Autodesk Inventor part; units mm, degrees
(part 2 of 5)
  arc A499 (38.985, 21.0742) -> (38.8363, 21.0784) centre (38.8363, 18.4135) ccw
  arc A500 (38.8363, 21.0784) -> (38.6875, 21.0742) centre (38.8363, 18.4135) ccw
  arc A501 (38.6875, 21.0742) -> (38.615, 21.0567) centre (38.6991, 20.8676) ccw
  arc A502 (38.615, 21.0567) -> (38.5792, 21.0205) centre (38.6435, 20.9926) ccw
  arc A503 (38.5792, 21.0205) -> (38.5663, 20.9584) centre (38.7225, 20.9584) ccw
  arc A504 (39.9268, 20.274) -> (39.9463, 20.2984) centre (39.9213, 20.2984) ccw
  arc A505 (39.8254, 20.2555) -> (39.9268, 20.274) centre (39.6443, 21.5339) ccw
  arc A506 (39.6897, 20.2426) -> (39.8254, 20.2555) centre (39.615, 21.7404) ccw
  arc A507 (39.5227, 20.2384) -> (39.6897, 20.2426) centre (39.5227, 23.5919) ccw
  arc A508 (39.3451, 20.242) -> (39.5227, 20.2384) centre (39.5227, 24.5793) ccw
  arc A509 (39.2206, 20.2542) -> (39.3451, 20.242) centre (39.3904, 21.3478) ccw
  arc A510 (39.1454, 20.2728) -> (39.2206, 20.2542) centre (39.2876, 20.686) ccw
  arc A511 (39.1363, 20.2984) -> (39.1454, 20.2728) centre (39.1511, 20.2893) ccw
  arc A512 (39.1697, 20.322) -> (39.1363, 20.2984) centre (39.1806, 20.271) ccw
  arc A513 (39.276, 20.3408) -> (39.1697, 20.322) centre (39.4953, 18.7927) ccw
  arc A514 (39.4091, 20.354) -> (39.276, 20.3408) centre (39.5025, 18.7417) ccw
  arc A515 (39.5598, 20.3584) -> (39.4091, 20.354) centre (39.5598, 17.7532) ccw
  arc A516 (39.7105, 20.3542) -> (39.5598, 20.3584) centre (39.5598, 17.6734) ccw
  arc A517 (39.8347, 20.3411) -> (39.7105, 20.3542) centre (39.6388, 19.0798) ccw
  arc A518 (39.9275, 20.3224) -> (39.8347, 20.3411) centre (39.6713, 19.289) ccw
  arc A519 (39.9463, 20.2984) -> (39.9275, 20.3224) centre (39.9216, 20.2984) ccw
  arc A520 (40.3232, 19.7911) -> (40.3363, 19.8184) centre (40.321, 19.8089) ccw
  arc A521 (40.1463, 19.7738) -> (40.3232, 19.7911) centre (39.8685, 23.525) ccw
  arc A522 (39.8917, 19.7619) -> (40.1463, 19.7738) centre (39.8016, 24.4273) ccw
  arc A523 (39.5263, 19.7584) -> (39.8917, 19.7619) centre (39.5263, 38.6953) ccw
  arc A524 (39.1609, 19.7619) -> (39.5263, 19.7584) centre (39.5263, 38.6953) ccw
  arc A525 (38.9062, 19.7738) -> (39.1609, 19.7619) centre (39.2509, 24.4273) ccw
  arc A526 (38.7294, 19.7911) -> (38.9062, 19.7738) centre (39.1841, 23.525) ccw
  arc A527 (38.7163, 19.8184) -> (38.7294, 19.7911) centre (38.7316, 19.8089) ccw
  arc A528 (38.7565, 19.8436) -> (38.7163, 19.8184) centre (38.7619, 19.7902) ccw
  arc A529 (38.9604, 19.8615) -> (38.7565, 19.8436) centre (39.5077, 12.4733) ccw
  arc A530 (39.2151, 19.8743) -> (38.9604, 19.8615) centre (39.3564, 14.5165) ccw
  arc A531 (39.5263, 19.8784) -> (39.2151, 19.8743) centre (39.5263, 8.073) ccw
  arc A532 (39.8375, 19.8743) -> (39.5263, 19.8784) centre (39.5263, 8.073) ccw
  arc A533 (40.0921, 19.8615) -> (39.8375, 19.8743) centre (39.6962, 14.5165) ccw
  arc A534 (40.2961, 19.8436) -> (40.0921, 19.8615) centre (39.5449, 12.4733) ccw
  arc A535 (40.3363, 19.8184) -> (40.2961, 19.8436) centre (40.2906, 19.7902) ccw
  arc A536 (40.3422, 19.3718) -> (40.3663, 19.3984) centre (40.3395, 19.3984) ccw
  arc A537 (40.1413, 19.3545) -> (40.3422, 19.3718) centre (39.6532, 26.1878) ccw
  arc A538 (39.8773, 19.3422) -> (40.1413, 19.3545) centre (39.7622, 24.661) ccw
  arc A539 (39.5263, 19.3384) -> (39.8773, 19.3422) centre (39.5263, 35.57) ccw
  arc A540 (39.1753, 19.3422) -> (39.5263, 19.3384) centre (39.5263, 35.57) ccw
  arc A541 (38.9113, 19.3545) -> (39.1753, 19.3422) centre (39.2903, 24.661) ccw
  arc A542 (38.7103, 19.3718) -> (38.9113, 19.3545) centre (39.3994, 26.1878) ccw
  arc A543 (38.6863, 19.3984) -> (38.7103, 19.3718) centre (38.713, 19.3984) ccw
  arc A544 (38.7103, 19.425) -> (38.6863, 19.3984) centre (38.713, 19.3984) ccw
  arc A545 (38.9113, 19.4423) -> (38.7103, 19.425) centre (39.3994, 12.609) ccw
  arc A546 (39.1753, 19.4546) -> (38.9113, 19.4423) centre (39.2903, 14.1358) ccw
  arc A547 (39.5263, 19.4584) -> (39.1753, 19.4546) centre (39.5263, 3.2268) ccw
  arc A548 (39.8773, 19.4546) -> (39.5263, 19.4584) centre (39.5263, 3.2268) ccw
  arc A549 (40.1413, 19.4423) -> (39.8773, 19.4546) centre (39.7622, 14.1358) ccw
  arc A550 (40.3422, 19.425) -> (40.1413, 19.4423) centre (39.6532, 12.609) ccw
  arc A551 (40.3663, 19.3984) -> (40.3422, 19.425) centre (40.3395, 19.3984) ccw
  arc A552 (39.1063, 18.1289) -> (39.0042, 18.0292) centre (40.3844, 16.7178) ccw
  arc A553 (39.0042, 18.0292) -> (38.9208, 17.9318) centre (39.9041, 17.1742) ccw
  arc A554 (38.9208, 17.9318) -> (38.862, 17.8473) centre (39.7541, 17.2897) ccw
  arc A555 (38.862, 17.8473) -> (38.8539, 17.8014) centre (38.9148, 17.8143) ccw
  arc A556 (38.8534, 17.7698) -> (38.8539, 17.8014) centre (38.7843, 17.7866) ccw
  arc A557 (38.8391, 17.7428) -> (38.8534, 17.7698) centre (38.793, 17.7845) ccw
  arc A558 (38.8129, 17.7247) -> (38.8391, 17.7428) centre (38.7881, 17.7889) ccw
  arc A559 (38.7789, 17.7184) -> (38.8129, 17.7247) centre (38.7789, 17.8128) ccw
  arc A560 (38.7349, 17.7356) -> (38.7789, 17.7184) centre (38.7789, 17.7833) ccw
  arc A561 (38.706, 17.7813) -> (38.7349, 17.7356) centre (38.806, 17.8126) ccw
  arc A562 (38.6904, 17.8667) -> (38.706, 17.7813) centre (39.0419, 17.8865) ccw
  arc A563 (38.6863, 18.014) -> (38.6904, 17.8667) centre (41.3006, 18.014) ccw
  arc A564 (38.6863, 18.014) -> (38.6816, 18.1645) centre (36.253, 18.014) ccw
  arc A565 (38.6816, 18.1645) -> (38.6646, 18.2541) centre (38.3197, 18.142) ccw
  arc A566 (38.6646, 18.2541) -> (38.6322, 18.3075) centre (38.5347, 18.2119) ccw
  arc A567 (38.6322, 18.3075) -> (38.5813, 18.337) centre (38.5534, 18.2302) ccw
  arc A568 (38.5813, 18.3478) -> (38.5813, 18.337) centre (38.5827, 18.3424) ccw
  arc A569 (38.6393, 18.3577) -> (38.5813, 18.3478) centre (38.6742, 17.9809) ccw
  arc A570 (38.7603, 18.3654) -> (38.6393, 18.3577) centre (38.8295, 16.3032) ccw
  arc A571 (38.9263, 18.369) -> (38.7603, 18.3654) centre (38.9968, 11.3177) ccw
  line L156 (38.9263, 18.369) -> (39.3763, 18.3735)
  line L157 (39.3763, 18.3735) -> (39.1063, 18.1289)
  arc A572 (40.71, 17.8434) -> (40.7396, 18.1384) centre (33.6679, 18.699) ccw
  arc A573 (40.6701, 17.7276) -> (40.71, 17.8434) centre (40.4206, 17.8785) ccw
  arc A574 (40.5987, 17.6831) -> (40.6701, 17.7276) centre (40.5905, 17.7757) ccw
  arc A575 (40.4691, 17.6911) -> (40.5987, 17.6831) centre (40.5604, 18.1178) ccw
  arc A576 (40.3093, 17.7285) -> (40.4691, 17.6911) centre (41.3948, 22.0136) ccw
  arc A577 (40.2608, 17.7568) -> (40.3093, 17.7285) centre (40.3342, 17.8266) ccw
  arc A578 (40.2559, 17.7953) -> (40.2608, 17.7568) centre (40.2846, 17.7794) ccw
  arc A579 (40.3036, 17.8651) -> (40.2559, 17.7953) centre (40.6516, 17.5763) ccw
  arc A580 (40.3036, 17.8651) -> (40.3314, 17.916) centre (40.1868, 17.962) ccw
  arc A581 (40.3314, 17.916) -> (40.3249, 17.9568) centre (40.2875, 17.9299) ccw
  arc A582 (40.3249, 17.9568) -> (40.2792, 17.9975) centre (40.2111, 17.875) ccw
  arc A583 (40.2792, 17.9975) -> (40.1665, 18.0556) centre (39.2902, 16.2179) ccw
  arc A584 (40.0747, 18.1066) -> (40.1665, 18.0556) centre (40.5332, 18.8245) ccw
  arc A585 (40.0105, 18.1596) -> (40.0747, 18.1066) centre (40.2585, 18.3945) ccw
  arc A586 (39.9736, 18.2142) -> (40.0105, 18.1596) centre (40.157, 18.2983) ccw
  arc A587 (39.9636, 18.2699) -> (39.9736, 18.2142) centre (40.0765, 18.2614) ccw
  arc A588 (39.9862, 18.329) -> (39.9636, 18.2699) centre (40.0742, 18.2615) ccw
  arc A589 (40.0362, 18.3614) -> (39.9862, 18.329) centre (40.057, 18.2747) ccw
  arc A590 (40.1372, 18.3726) -> (40.0362, 18.3614) centre (40.1311, 17.9654) ccw
  arc A591 (40.3642, 18.3658) -> (40.1372, 18.3726) centre (40.0207, 10.6454) ccw
  line L158 (40.3642, 18.3658) -> (40.7563, 18.3484)
  line L159 (40.7563, 18.3484) -> (40.7396, 18.1384)
  arc A592 (39.7374, 17.7553) -> (39.7363, 17.7784) centre (39.716, 17.7659) ccw
  arc A593 (39.7177, 17.7356) -> (39.7374, 17.7553) centre (39.6982, 17.7747) ccw
  arc A594 (39.6756, 17.7225) -> (39.7177, 17.7356) centre (39.6568, 17.8575) ccw
  arc A595 (39.6163, 17.7184) -> (39.6756, 17.7225) centre (39.6163, 18.149) ccw
  arc A596 (39.557, 17.7225) -> (39.6163, 17.7184) centre (39.6163, 18.149) ccw
  arc A597 (39.5148, 17.7356) -> (39.557, 17.7225) centre (39.5758, 17.8575) ccw
  arc A598 (39.4952, 17.7553) -> (39.5148, 17.7356) centre (39.5344, 17.7747) ccw
  arc A599 (39.4963, 17.7784) -> (39.4952, 17.7553) centre (39.5166, 17.7659) ccw
  arc A600 (39.5166, 17.8014) -> (39.4963, 17.7784) centre (39.5733, 17.7308) ccw
  arc A601 (39.5468, 17.8208) -> (39.5166, 17.8014) centre (39.6223, 17.6699) ccw
  arc A602 (39.5818, 17.8339) -> (39.5468, 17.8208) centre (39.6278, 17.6589) ccw
  arc A603 (39.6163, 17.8384) -> (39.5818, 17.8339) centre (39.6163, 17.7027) ccw
  arc A604 (39.6507, 17.8339) -> (39.6163, 17.8384) centre (39.6163, 17.7027) ccw
  arc A605 (39.6857, 17.8208) -> (39.6507, 17.8339) centre (39.6048, 17.6589) ccw
  arc A606 (39.716, 17.8014) -> (39.6857, 17.8208) centre (39.6103, 17.6699) ccw
  arc A607 (39.7363, 17.7784) -> (39.716, 17.8014) centre (39.6593, 17.7308) ccw
  arc A608 (24.9198, 18.924) -> (24.9355, 19.7434) centre (-73.7017, 21.2341) ccw
  arc A609 (24.8971, 18.5938) -> (24.9198, 18.924) centre (21.24, 19.0102) ccw
  arc A610 (24.849, 18.3735) -> (24.8971, 18.5938) centre (23.794, 18.7194) ccw
  arc A611 (24.7528, 18.1384) -> (24.849, 18.3735) centre (23.1606, 18.9271) ccw
  arc A612 (24.6847, 18.0044) -> (24.7528, 18.1384) centre (18.3822, 21.294) ccw
  arc A613 (24.6151, 17.8746) -> (24.6847, 18.0044) centre (18.8834, 21.0324) ccw
  arc A614 (24.5527, 17.7643) -> (24.6151, 17.8746) centre (19.4498, 20.7203) ccw
  arc A615 (24.5134, 17.7038) -> (24.5527, 17.7643) centre (23.9472, 18.1151) ccw
  arc A616 (24.5134, 17.7038) -> (24.4842, 17.6387) centre (24.654, 17.6017) ccw
  arc A617 (24.4842, 17.6387) -> (24.4906, 17.578) centre (24.5791, 17.618) ccw
  arc A618 (24.4906, 17.578) -> (24.5398, 17.503) centre (24.7533, 17.6967) ccw
  arc A619 (24.5398, 17.503) -> (24.6623, 17.3744) centre (27.2389, 19.951) ccw
  arc A620 (24.6623, 17.3744) -> (24.8458, 17.2238) centre (25.5185, 18.2306) ccw
  arc A621 (24.8458, 17.2238) -> (24.9744, 17.2094) centre (24.9241, 17.3409) ccw
  arc A622 (24.9744, 17.2094) -> (25.0949, 17.3087) centre (24.8867, 17.4385) ccw
  arc A623 (25.0949, 17.3087) -> (25.2625, 17.6043) centre (21.6467, 19.4587) ccw
  arc A624 (25.2625, 17.6043) -> (25.4059, 17.9657) centre (23.4592, 18.5292) ccw
  arc A625 (25.4059, 17.9657) -> (25.4906, 18.3747) centre (22.8196, 18.7143) ccw
  arc A626 (25.4906, 18.3747) -> (25.5337, 18.9364) centre (19.8759, 19.0886) ccw
  arc A627 (25.5337, 18.9364) -> (25.5459, 19.8334) centre (-8.1742, 19.8433) ccw
  line L160 (25.5459, 19.8334) -> (25.5463, 21.0184)
  line L161 (25.5463, 21.0184) -> (25.2505, 21.0184)
  line L162 (25.2505, 21.0184) -> (24.9548, 21.0184)
  line L163 (24.9548, 21.0184) -> (24.9355, 19.7434)
  line L164 (26.2063, 19.2484) -> (26.2063, 17.5384)
  line L165 (26.2063, 17.5384) -> (26.5063, 17.5384)
  line L166 (26.5063, 17.5384) -> (26.8063, 17.5384)
  line L167 (26.8063, 17.5384) -> (26.8063, 19.2484)
  line L168 (26.8063, 19.2484) -> (26.8063, 20.9584)
  line L169 (26.8063, 20.9584) -> (26.5063, 20.9584)
  line L170 (26.5063, 20.9584) -> (26.2063, 20.9584)
  line L171 (26.2063, 20.9584) -> (26.2063, 19.2484)
  arc A628 (63.6763, 20.8683) -> (63.3127, 20.6476) centre (64.0233, 19.8867) ccw
  arc A629 (63.3127, 20.6476) -> (63.0596, 20.2962) centre (64.0749, 19.8316) ccw
  arc A630 (63.0596, 20.2962) -> (62.9127, 19.7889) centre (64.694, 19.5482) ccw
  arc A631 (62.9127, 19.7889) -> (62.8663, 19.0982) centre (68.0247, 19.0982) ccw
  arc A632 (62.8663, 19.0982) -> (62.8863, 18.5942) centre (69.226, 19.0982) ccw
  arc A633 (62.8863, 18.5942) -> (62.9514, 18.2296) centre (64.7853, 18.7452) ccw
  arc A634 (62.9514, 18.2296) -> (63.0717, 17.9452) centre (64.1319, 18.5615) ccw
  arc A635 (63.0717, 17.9452) -> (63.2603, 17.6964) centre (64.1797, 18.5892) ccw
  arc A636 (63.2603, 17.6964) -> (63.5324, 17.4875) centre (64.1103, 18.5219) ccw
  arc A637 (63.5324, 17.4875) -> (63.8374, 17.3808) centre (63.9905, 18.3075) ccw
  arc A638 (63.8374, 17.3808) -> (64.1613, 17.3835) centre (63.9915, 18.3131) ccw
  arc A639 (64.1613, 17.3835) -> (64.4886, 17.4934) centre (63.9438, 18.5736) ccw
  arc A640 (64.4886, 17.4934) -> (64.629, 17.5768) centre (63.9526, 18.5563) ccw
  arc A641 (64.629, 17.5768) -> (64.736, 17.6688) centre (64.2487, 18.1275) ccw
  arc A642 (64.736, 17.6688) -> (64.8288, 17.7883) centre (64.1563, 18.2144) ccw
  arc A643 (64.8288, 17.7883) -> (64.9262, 17.9584) centre (62.9718, 18.965) ccw
  arc A644 (64.9262, 17.9584) -> (65.0181, 18.1537) centre (62.2593, 19.3319) ccw
  arc A645 (65.0181, 18.1537) -> (65.0618, 18.2958) centre (64.3683, 18.4313) ccw
  arc A646 (65.0618, 18.2958) -> (65.0749, 18.4442) centre (64.3619, 18.4325) ccw
  arc A647 (65.0749, 18.4442) -> (65.0637, 18.6617) centre (61.9854, 18.3934) ccw
  arc A648 (65.0637, 18.6617) -> (64.9964, 19.0331) centre (63.0214, 18.4837) ccw
  arc A649 (64.9964, 19.0331) -> (64.8656, 19.3269) centre (63.9416, 18.7396) ccw
  arc A650 (64.8656, 19.3269) -> (64.6691, 19.5455) centre (64.1157, 18.8503) ccw
  arc A651 (64.6691, 19.5455) -> (64.4074, 19.6944) centre (64.062, 18.7828) ccw
  arc A652 (64.4074, 19.6944) -> (64.2257, 19.7447) centre (64.0447, 18.7371) ccw
  arc A653 (64.2257, 19.7447) -> (64.065, 19.7496) centre (64.1286, 19.2044) ccw
  arc A654 (64.065, 19.7496) -> (63.8958, 19.7072) centre (64.1432, 19.0792) ccw
  arc A655 (63.8958, 19.7072) -> (63.6852, 19.6101) centre (64.6466, 17.8021) ccw
  arc A656 (63.4852, 19.5106) -> (63.6852, 19.6101) centre (61.7458, 23.2576) ccw
  arc A657 (63.4283, 19.5227) -> (63.4852, 19.5106) centre (63.4648, 19.5545) ccw
  arc A658 (63.4115, 19.588) -> (63.4283, 19.5227) centre (63.4849, 19.572) ccw
  arc A659 (63.4736, 19.8527) -> (63.4115, 19.588) centre (71.5899, 17.809) ccw
  arc A660 (63.6474, 20.197) -> (63.4736, 19.8527) centre (64.3277, 19.6376) ccw
  arc A661 (63.9372, 20.391) -> (63.6474, 20.197) centre (64.1141, 19.8132) ccw
  arc A662 (64.229, 20.3658) -> (63.9372, 20.391) centre (64.0518, 20.0166) ccw
  arc A663 (64.4277, 20.1447) -> (64.229, 20.3658) centre (64.0425, 19.9983) ccw
  arc A664 (64.4277, 20.1447) -> (64.4693, 20.0675) centre (64.7431, 20.2647) ccw
  arc A665 (64.4693, 20.0675) -> (64.5224, 20.0244) centre (64.5751, 20.1437) ccw
  arc A666 (64.5224, 20.0244) -> (64.6057, 20.0037) centre (64.623, 20.2522) ccw
  arc A667 (64.6057, 20.0037) -> (64.7588, 19.9984) centre (64.7588, 22.1934) ccw
  arc A668 (64.7588, 19.9984) -> (64.928, 20.0015) centre (64.7588, 24.6481) ccw
  arc A669 (64.928, 20.0015) -> (64.9872, 20.0185) centre (64.9234, 20.129) ccw
  arc A670 (64.9872, 20.0185) -> (65.0071, 20.0559) centre (64.9672, 20.0532) ccw
  arc A671 (65.0071, 20.0559) -> (64.9927, 20.1334) centre (64.6659, 20.0326) ccw
  arc A672 (64.9927, 20.1334) -> (64.8784, 20.4076) centre (63.5101, 19.676) ccw
  arc A673 (64.8784, 20.4076) -> (64.7207, 20.632) centre (63.8809, 19.8743) ccw
  arc A674 (64.7207, 20.632) -> (64.5258, 20.7979) centre (63.997, 19.9791) ccw
  arc A675 (64.5258, 20.7979) -> (64.3013, 20.8998) centre (64.0693, 20.091) ccw
  arc A676 (64.3013, 20.8998) -> (64.126, 20.9419) centre (63.7321, 18.9152) ccw
  arc A677 (64.126, 20.9419) -> (63.9999, 20.9509) centre (64.0262, 20.4286) ccw
  arc A678 (63.9999, 20.9509) -> (63.8696, 20.9295) centre (64.0297, 20.3597) ccw
  arc A679 (63.8696, 20.9295) -> (63.6763, 20.8683) centre (64.7023, 17.9664) ccw
  arc A680 (64.5137, 18.8064) -> (64.3656, 19.051) centre (64.1001, 18.7232) ccw
  arc A681 (64.5184, 18.4478) -> (64.5137, 18.8064) centre (63.5595, 18.6144) ccw
  arc A682 (64.3931, 18.1122) -> (64.5184, 18.4478) centre (63.5609, 18.6142) ccw
  arc A683 (64.1713, 17.9325) -> (64.3931, 18.1122) centre (64.0338, 18.3289) ccw
  arc A684 (63.9839, 17.9028) -> (64.1713, 17.9325) centre (63.9945, 18.4422) ccw
  arc A685 (63.8154, 17.9453) -> (63.9839, 17.9028) centre (63.9914, 18.2879) ccw
  arc A686 (63.6677, 18.0636) -> (63.8154, 17.9453) centre (64.0322, 18.3673) ccw
  arc A687 (63.5413, 18.2562) -> (63.6677, 18.0636) centre (64.4475, 18.7133) ccw
  arc A688 (63.438, 18.4936) -> (63.5413, 18.2562) centre (65.5813, 19.2851) ccw
  arc A689 (63.4179, 18.6498) -> (63.438, 18.4936) centre (63.7673, 18.6152) ccw
  arc A690 (63.4693, 18.7873) -> (63.4179, 18.6498) centre (63.7032, 18.6216) ccw
  arc A691 (63.6103, 18.9544) -> (63.4693, 18.7873) centre (64.5255, 18.0392) ccw
  arc A692 (63.7948, 19.0929) -> (63.6103, 18.9544) centre (64.1882, 18.3765) ccw
  arc A693 (63.9941, 19.1578) -> (63.7948, 19.0929) centre (64.0655, 18.6) ccw
  arc A694 (64.19, 19.1426) -> (63.9941, 19.1578) centre (64.0556, 18.6774) ccw
  arc A695 (64.3656, 19.051) -> (64.19, 19.1426) centre (64.0515, 18.6631) ccw
  line L172 (20.0863, 20.6284) -> (20.0863, 20.3584)
  line L173 (20.0863, 20.3584) -> (22.0663, 20.3584)
  line L174 (22.0663, 20.3584) -> (24.0463, 20.3584)
  line L175 (24.0463, 20.3584) -> (24.0463, 20.6284)
  line L176 (24.0463, 20.6284) -> (24.0463, 20.8984)
  line L177 (24.0463, 20.8984) -> (22.0663, 20.8984)
  line L178 (22.0663, 20.8984) -> (20.0863, 20.8984)
  line L179 (20.0863, 20.8984) -> (20.0863, 20.6284)
  line L180 (28.9663, 19.0084) -> (28.9663, 17.1184)
  line L181 (28.9663, 17.1184) -> (29.2663, 17.1184)
  arc A696 (29.2663, 17.1184) -> (29.4139, 17.1226) centre (29.2663, 19.7435) ccw
  arc A697 (29.4139, 17.1226) -> (29.5013, 17.1379) centre (29.3926, 17.5) ccw
  arc A698 (29.5013, 17.1379) -> (29.5486, 17.166) centre (29.4686, 17.2468) ccw
  arc A699 (29.5486, 17.166) -> (29.5663, 17.2084) centre (29.5066, 17.2084) ccw
  arc A700 (29.6112, 17.2599) -> (29.5663, 17.2084) centre (29.6182, 17.2084) ccw
  arc A701 (29.8463, 17.2825) -> (29.6112, 17.2599) centre (30.015, 14.3025) ccw
  arc A702 (30.2603, 17.2956) -> (29.8463, 17.2825) centre (30.3124, 9.0472) ccw
  arc A703 (31.1563, 17.2984) -> (30.2603, 17.2956) centre (31.1563, -124.4743) ccw
  line L182 (31.1563, 17.2984) -> (32.7463, 17.2984)
  line L183 (32.7463, 17.2984) -> (32.7463, 17.5984)
  line L184 (32.7463, 17.5984) -> (32.7463, 17.8984)
  line L185 (32.7463, 17.8984) -> (31.1563, 17.8984)
  line L186 (31.1563, 17.8984) -> (29.5663, 17.8984)
  line L187 (29.5663, 17.8984) -> (29.5663, 19.1284)
  line L188 (29.5663, 19.1284) -> (29.5663, 20.3584)
  line L189 (29.5663, 20.3584) -> (30.615, 20.3584)
  line L190 (30.615, 20.3584) -> (31.6637, 20.3584)
  line L191 (31.6637, 20.3584) -> (31.5921, 20.1934)
  arc A704 (31.4918, 19.9886) -> (31.5921, 20.1934) centre (29.3306, 21.1746) ccw
  arc A705 (31.3683, 19.7835) -> (31.4918, 19.9886) centre (28.8728, 21.4258) ccw
  arc A706 (31.2462, 19.6082) -> (31.3683, 19.7835) centre (27.9397, 22.0399) ccw
  arc A707 (31.1874, 19.5784) -> (31.2462, 19.6082) centre (31.1874, 19.6514) ccw
  arc A708 (31.1493, 19.5883) -> (31.1874, 19.5784) centre (31.1874, 19.6565) ccw
  arc A709 (31.0112, 19.667) -> (31.1493, 19.5883) centre (35.7759, 27.8726) ccw
  arc A710 (30.8492, 19.7644) -> (31.0112, 19.667) centre (34.0652, 24.9265) ccw
  arc A711 (30.668, 19.88) -> (30.8492, 19.7644) centre (36.2119, 28.3724) ccw
  line L192 (30.668, 19.88) -> (30.2061, 20.1815)
  line L193 (30.2061, 20.1815) -> (30.0362, 20.0187)
  arc A712 (30.0362, 20.0187) -> (29.9099, 19.8825) centre (31.1185, 18.8891) ccw
  arc A713 (29.9099, 19.8825) -> (29.8755, 19.7907) centre (30.0269, 19.7863) ccw
  arc A714 (29.8755, 19.7907) -> (29.9101, 19.7161) centre (29.9677, 19.788) ccw
  arc A715 (29.9101, 19.7161) -> (30.0255, 19.6451) centre (30.2532, 20.1448) ccw
  arc A716 (30.1082, 19.603) -> (30.0255, 19.6451) centre (29.5798, 18.6669) ccw
  arc A717 (30.2349, 19.5295) -> (30.1082, 19.603) centre (27.0585, 14.2001) ccw
  arc A718 (30.3767, 19.4427) -> (30.2349, 19.5295) centre (26.6613, 13.5337) ccw
  arc A719 (30.5147, 19.3536) -> (30.3767, 19.4427) centre (26.8343, 13.8088) ccw
  line L194 (30.5147, 19.3536) -> (30.8446, 19.1346)
  line L195 (30.8446, 19.1346) -> (30.6118, 18.9333)
  arc A720 (30.4985, 18.8446) -> (30.6118, 18.9333) centre (29.6402, 20.0573) ccw
  arc A721 (30.3479, 18.7435) -> (30.4985, 18.8446) centre (28.3613, 21.8645) ccw
  arc A722 (30.1869, 18.6464) -> (30.3479, 18.7435) centre (28.2706, 22.0069) ccw
  arc A723 (30.0402, 18.5695) -> (30.1869, 18.6464) centre (29.027, 20.6804) ccw
  line L196 (30.0402, 18.5695) -> (29.7013, 18.4069)
  line L197 (29.7013, 18.4069) -> (29.9021, 18.1746)
  arc A724 (29.9021, 18.1746) -> (30.0332, 18.03) centre (33.034, 20.882) ccw
  arc A725 (30.0332, 18.03) -> (30.1022, 17.9841) centre (30.1687, 18.1589) ccw
  arc A726 (30.1022, 17.9841) -> (30.174, 17.9807) centre (30.1433, 18.092) ccw
  arc A727 (30.174, 17.9807) -> (30.2988, 18.0236) centre (29.8886, 19.0139) ccw
  arc A728 (30.2988, 18.0236) -> (30.3989, 18.0734) centre (29.9889, 18.7716) ccw
  arc A729 (30.3989, 18.0734) -> (30.5485, 18.1652) centre (28.0866, 22.0113) ccw
  arc A730 (30.5485, 18.1652) -> (30.7142, 18.2758) centre (27.7646, 22.5143) ccw
  arc A731 (30.7142, 18.2758) -> (30.8737, 18.3916) centre (27.8947, 22.3274) ccw
  arc A732 (31.0229, 18.5015) -> (30.8737, 18.3916) centre (35.0971, 12.8117) ccw
  arc A733 (31.1578, 18.5941) -> (31.0229, 18.5015) centre (33.5011, 15.0406) ccw
  arc A734 (31.2727, 18.6681) -> (31.1578, 18.5941) centre (34.4502, 13.6012) ccw
  arc A735 (31.3086, 18.6784) -> (31.2727, 18.6681) centre (31.3086, 18.6107) ccw
  arc A736 (31.3444, 18.667) -> (31.3086, 18.6784) centre (31.3086, 18.6166) ccw
  arc A737 (31.4627, 18.5813) -> (31.3444, 18.667) centre (27.5185, 13.2635) ccw
  arc A738 (31.6009, 18.4745) -> (31.4627, 18.5813) centre (28.7887, 14.976) ccw
  arc A739 (31.7543, 18.3479) -> (31.6009, 18.4745) centre (26.8872, 12.6106) ccw
  line L198 (31.7543, 18.3479) -> (32.1439, 18.0174)
  line L199 (32.1439, 18.0174) -> (32.3028, 18.2575)
  arc A740 (32.3028, 18.2575) -> (32.4025, 18.4388) centre (31.2466, 18.9564) ccw
  arc A741 (32.4025, 18.4388) -> (32.4029, 18.5505) centre (32.2769, 18.4951) ccw
  arc A742 (32.4029, 18.5505) -> (32.3173, 18.6635) centre (32.1229, 18.4273) ccw
  arc A743 (32.3173, 18.6635) -> (32.0209, 18.8984) centre (25.8668, 10.8287) ccw
  arc A744 (31.908, 18.988) -> (32.0209, 18.8984) centre (34.2667, 21.8433) ccw
  arc A745 (31.8128, 19.0713) -> (31.908, 18.988) centre (33.3116, 20.6872) ccw
  arc A746 (31.7379, 19.1435) -> (31.8128, 19.0713) centre (33.6704, 21.074) ccw
  arc A747 (31.7263, 19.1716) -> (31.7379, 19.1435) centre (31.7661, 19.1716) ccw
  arc A748 (31.7341, 19.203) -> (31.7263, 19.1716) centre (31.7929, 19.1716) ccw
  arc A749 (31.7863, 19.2982) -> (31.7341, 19.203) centre (35.7961, 17.0386) ccw
  arc A750 (31.8524, 19.4105) -> (31.7863, 19.2982) centre (34.8193, 17.5891) ccw
  arc A751 (31.9307, 19.5343) -> (31.8524, 19.4105) centre (36.6008, 16.4954) ccw
  arc A752 (31.9307, 19.5343) -> (32.1232, 19.8479) centre (26.0617, 23.3533) ccw
  arc A753 (32.1232, 19.8479) -> (32.1773, 20.0103) centre (31.7547, 20.061) ccw
  arc A754 (32.1773, 20.0103) -> (32.143, 20.1263) centre (32.0256, 20.0285) ccw
  arc A755 (32.143, 20.1263) -> (32.0149, 20.2369) centre (31.7458, 19.7954) ccw
  line L200 (32.0149, 20.2369) -> (31.8163, 20.3579)
  line L201 (31.8163, 20.3579) -> (32.2213, 20.3582)
  line L202 (32.2213, 20.3582) -> (32.6263, 20.3584)
  line L203 (32.6263, 20.3584) -> (32.6263, 20.6284)
  line L204 (32.6263, 20.6284) -> (32.6263, 20.8984)
  line L205 (32.6263, 20.8984) -> (30.7963, 20.8984)
  line L206 (30.7963, 20.8984) -> (28.9663, 20.8984)
  line L207 (28.9663, 20.8984) -> (28.9663, 19.0084)
  line L208 (41.9263, 20.6306) -> (41.9263, 20.3627)
  line L209 (41.9263, 20.3627) -> (42.5113, 20.3456)
  line L210 (42.5113, 20.3456) -> (43.0963, 20.3284)
  line L211 (43.0963, 20.3284) -> (43.0963, 20.1484)
  line L212 (43.0963, 20.1484) -> (43.0963, 19.9684)
  line L213 (43.0963, 19.9684) -> (42.6013, 19.951)
  line L214 (42.6013, 19.951) -> (42.1063, 19.9335)
  line L215 (42.1063, 19.9335) -> (42.1063, 18.556)
  line L216 (42.1063, 18.556) -> (42.1063, 17.1784)
  line L217 (42.1063, 17.1784) -> (42.4063, 17.1784)
  arc A756 (42.4063, 17.1784) -> (42.5213, 17.1827) centre (42.4063, 18.7068) ccw
  arc A757 (42.5213, 17.1827) -> (42.6182, 17.196) centre (42.461, 17.982) ccw
  arc A758 (42.6182, 17.196) -> (42.6894, 17.215) centre (42.503, 17.7717) ccw
  arc A759 (42.6894, 17.215) -> (42.7063, 17.2384) centre (42.6816, 17.2384) ccw
  arc A760 (42.732, 17.2659) -> (42.7063, 17.2384) centre (42.7338, 17.2384) ccw
  arc A761 (43.0213, 17.2826) -> (42.732, 17.2659) centre (43.9239, -0.7703) ccw
  arc A762 (43.3959, 17.2947) -> (43.0213, 17.2826) centre (43.5482, 6.7434) ccw
  arc A763 (43.9063, 17.2984) -> (43.3959, 17.2947) centre (43.9063, -18.0563) ccw
  arc A764 (44.4166, 17.2947) -> (43.9063, 17.2984) centre (43.9063, -18.0563) ccw
  arc A765 (44.7913, 17.2826) -> (44.4166, 17.2947) centre (44.2643, 6.7434) ccw
  arc A766 (45.0806, 17.2659) -> (44.7913, 17.2826) centre (43.8886, -0.7703) ccw
  arc A767 (45.1063, 17.2384) -> (45.0806, 17.2659) centre (45.0788, 17.2384) ccw
  arc A768 (45.1063, 17.2384) -> (45.1231, 17.215) centre (45.1309, 17.2384) ccw
  arc A769 (45.1231, 17.215) -> (45.1944, 17.196) centre (45.3095, 17.7717) ccw
  arc A770 (45.1944, 17.196) -> (45.2913, 17.1827) centre (45.3516, 17.982) ccw
  arc A771 (45.2913, 17.1827) -> (45.4063, 17.1784) centre (45.4063, 18.7068) ccw
  line L218 (45.4063, 17.1784) -> (45.7063, 17.1784)
  line L219 (45.7063, 17.1784) -> (45.7063, 18.5584)
  line L220 (45.7063, 18.5584) -> (45.7063, 19.9384)
  line L221 (45.7063, 19.9384) -> (45.1363, 19.9384)
  line L222 (45.1363, 19.9384) -> (44.5663, 19.9384)
  line L223 (44.5663, 19.9384) -> (44.5663, 20.1484)
  line L224 (44.5663, 20.1484) -> (44.5663, 20.3584)
  line L225 (44.5663, 20.3584) -> (45.1963, 20.3584)
  line L226 (45.1963, 20.3584) -> (45.8263, 20.3584)
  line L227 (45.8263, 20.3584) -> (45.8263, 20.6284)
  line L228 (45.8263, 20.6284) -> (45.8263, 20.8984)
  line L229 (45.8263, 20.8984) -> (43.8763, 20.8984)
  line L230 (43.8763, 20.8984) -> (41.9263, 20.8984)
  line L231 (41.9263, 20.8984) -> (41.9263, 20.6306)
  arc A772 (43.962, 20.0236) -> (43.9663, 20.1442) centre (42.2747, 20.1442) ccw
  arc A773 (43.9432, 19.9701) -> (43.962, 20.0236) centre (43.8544, 20.0313) ccw
  arc A774 (43.9047, 19.9475) -> (43.9432, 19.9701) centre (43.8997, 20.0001) ccw
  arc A775 (43.8319, 19.9492) -> (43.9047, 19.9475) centre (43.8755, 20.255) ccw
  arc A776 (43.7102, 20.0218) -> (43.8319, 19.9492) centre (43.8579, 20.1312) ccw
  arc A777 (43.6649, 20.1661) -> (43.7102, 20.0218) centre (43.8955, 20.1591) ccw
  arc A778 (43.7195, 20.3026) -> (43.6649, 20.1661) centre (43.8792, 20.1596) ccw
  arc A779 (43.8444, 20.3584) -> (43.7195, 20.3026) centre (43.8444, 20.1908) ccw
  arc A780 (43.906, 20.3478) -> (43.8444, 20.3584) centre (43.8444, 20.1741) ccw
  arc A781 (43.9427, 20.317) -> (43.906, 20.3478) centre (43.8831, 20.2831) ccw
  arc A782 (43.9614, 20.2571) -> (43.9427, 20.317) centre (43.8151, 20.2444) ccw
  arc A783 (43.9663, 20.1442) -> (43.9614, 20.2571) centre (42.6554, 20.1442) ccw
  arc A784 (43.0444, 19.0901) -> (43.0663, 19.2425) centre (42.5249, 19.2425) ccw
  arc A785 (42.9749, 18.8993) -> (43.0444, 19.0901) centre (41.5178, 19.5379) ccw
  arc A786 (42.8832, 18.7216) -> (42.9749, 18.8993) centre (41.5295, 19.5328) ccw
  arc A787 (42.7908, 18.6138) -> (42.8832, 18.7216) centre (42.5213, 18.9385) ccw
  arc A788 (42.7497, 18.6054) -> (42.7908, 18.6138) centre (42.7624, 18.648) ccw
  arc A789 (42.7218, 18.635) -> (42.7497, 18.6054) centre (42.7613, 18.6444) ccw
  arc A790 (42.7089, 18.7355) -> (42.7218, 18.635) centre (43.1926, 18.7463) ccw
  arc A791 (42.7063, 18.9711) -> (42.7089, 18.7355) centre (53.2102, 18.9711) ccw
  line L232 (42.7063, 18.9711) -> (42.7063, 19.3984)
  line L233 (42.7063, 19.3984) -> (42.8863, 19.3984)
  arc A792 (42.9841, 19.3925) -> (42.8863, 19.3984) centre (42.8863, 18.5848) ccw
  arc A793 (43.034, 19.3704) -> (42.9841, 19.3925) centre (42.9729, 19.2999) ccw
  arc A794 (43.059, 19.3262) -> (43.034, 19.3704) centre (42.9843, 19.3131) ccw
  arc A795 (43.0663, 19.2425) -> (43.059, 19.3262) centre (42.5813, 19.2425) ccw
  arc A796 (43.9663, 18.9484) -> (43.9712, 18.7024) centre (50.1205, 18.9484) ccw
  arc A797 (43.9712, 18.7024) -> (43.9897, 18.5584) centre (44.7974, 18.7354) ccw
  arc A798 (43.9897, 18.5584) -> (44.0274, 18.4586) centre (44.3499, 18.6374) ccw
  arc A799 (44.0274, 18.4586) -> (44.0925, 18.3722) centre (44.3675, 18.6471) ccw
  arc A800 (44.0925, 18.3722) -> (44.1794, 18.3058) centre (44.3845, 18.6642) ccw
  arc A801 (44.1794, 18.3058) -> (44.2736, 18.2714) centre (44.3264, 18.5625) ccw
  arc A802 (44.2736, 18.2714) -> (44.4107, 18.2601) centre (44.4001, 18.97) ccw
  arc A803 (44.4107, 18.2601) -> (44.6653, 18.2685) centre (44.3034, 25.4357) ccw
  line L234 (44.6653, 18.2685) -> (45.1119, 18.291)
  line L235 (45.1119, 18.291) -> (45.0941, 18.0797)
  line L236 (45.0941, 18.0797) -> (45.0763, 17.8684)
  line L237 (45.0763, 17.8684) -> (43.8913, 17.8521)
  line L238 (43.8913, 17.8521) -> (42.7063, 17.8359)
  line L239 (42.7063, 17.8359) -> (42.708, 18.1221)
  line L240 (42.708, 18.1221) -> (42.7098, 18.4084)
  line L241 (42.7098, 18.4084) -> (42.8959, 18.2037)
  arc A804 (42.8959, 18.2037) -> (43.0463, 18.0703) centre (43.5878, 18.8326) ccw
  arc A805 (43.0463, 18.0703) -> (43.1591, 18.0541) centre (43.1185, 18.1719) ccw
  arc A806 (43.1591, 18.0541) -> (43.2734, 18.1382) centre (43.0813, 18.2795) ccw
  arc A807 (43.2734, 18.1382) -> (43.4465, 18.3937) centre (40.0767, 20.4902) ccw
  arc A808 (43.4465, 18.3937) -> (43.5255, 18.5393) centre (42.2624, 19.1303) ccw
  arc A809 (43.5255, 18.5393) -> (43.5841, 18.6891) centre (42.4009, 19.0655) ccw
  arc A810 (43.5841, 18.6891) -> (43.6247, 18.851) centre (42.302, 19.097) ccw
  arc A811 (43.6247, 18.851) -> (43.6498, 19.0328) centre (41.6931, 19.2102) ccw
  arc A812 (43.6734, 19.2507) -> (43.6498, 19.0328) centre (49.955, 18.4611) ccw
  arc A813 (43.6999, 19.3412) -> (43.6734, 19.2507) centre (43.9662, 19.2138) ccw
  arc A814 (43.7455, 19.3835) -> (43.6999, 19.3412) centre (43.7763, 19.3047) ccw
  arc A815 (43.8246, 19.3984) -> (43.7455, 19.3835) centre (43.8246, 19.1809) ccw
  arc A816 (43.905, 19.3818) -> (43.8246, 19.3984) centre (43.8246, 19.1955) ccw
  arc A817 (43.9466, 19.3358) -> (43.905, 19.3818) centre (43.8755, 19.3134) ccw
  arc A818 (43.9633, 19.2338) -> (43.9466, 19.3358) centre (43.5985, 19.2262) ccw
  arc A819 (43.9663, 18.9484) -> (43.9633, 19.2338) centre (30.217, 18.9484) ccw
  arc A820 (45.0993, 18.9989) -> (45.1063, 19.1584) centre (43.2893, 19.1584) ccw
  arc A821 (45.0685, 18.9346) -> (45.0993, 18.9989) centre (44.9981, 19.0079) ccw
  arc A822 (45.017, 18.9289) -> (45.0685, 18.9346) centre (45.0391, 18.9652) ccw
  arc A823 (44.9345, 18.9934) -> (45.017, 18.9289) centre (45.2496, 19.3116) ccw
  arc A824 (44.9345, 18.9934) -> (44.8933, 19.0268) centre (44.7482, 18.8052) ccw
  arc A825 (44.8933, 19.0268) -> (44.8621, 19.0325) centre (44.8709, 18.9926) ccw
  arc A826 (44.8621, 19.0325) -> (44.8333, 19.0142) centre (44.873, 18.9834) ccw
  arc A827 (44.8333, 19.0142) -> (44.7996, 18.9634) centre (45.1659, 18.7567) ccw
  arc A828 (44.7162, 18.8637) -> (44.7996, 18.9634) centre (44.4879, 19.1392) ccw
  arc A829 (44.6394, 18.8607) -> (44.7162, 18.8637) centre (44.6759, 18.9123) ccw
  arc A830 (44.5827, 18.9493) -> (44.6394, 18.8607) centre (44.72, 18.9747) ccw
  arc A831 (44.5663, 19.1284) -> (44.5827, 18.9493) centre (45.5506, 19.1284) ccw
  line L242 (44.5663, 19.1284) -> (44.5663, 19.3984)
  line L243 (44.5663, 19.3984) -> (44.8363, 19.3984)
  line L244 (44.8363, 19.3984) -> (45.1063, 19.3984)
  line L245 (45.1063, 19.3984) -> (45.1063, 19.1584)
  arc A832 (47.282, 20.556) -> (47.3563, 20.6732) centre (46.5325, 21.1129) ccw
  arc A833 (47.2034, 20.4762) -> (47.282, 20.556) centre (46.9572, 20.7973) ccw
  arc A834 (47.1011, 20.4167) -> (47.2034, 20.4762) centre (46.9203, 20.8455) ccw
  arc A835 (46.9513, 20.3628) -> (47.1011, 20.4167) centre (46.5246, 21.7837) ccw
  arc A836 (46.9513, 20.3628) -> (46.7812, 20.3062) centre (47.8126, 17.4944) ccw
  arc A837 (46.7812, 20.3062) -> (46.7092, 20.2601) centre (46.8496, 20.1196) ccw
  arc A838 (46.7092, 20.2601) -> (46.6759, 20.1955) centre (46.7932, 20.1761) ccw
  arc A839 (46.6759, 20.1955) -> (46.6663, 20.0778) centre (47.3874, 20.0778) ccw
  line L246 (46.6663, 20.0778) -> (46.6663, 19.8784)
  line L247 (46.6663, 19.8784) -> (46.9963, 19.8784)
  line L248 (46.9963, 19.8784) -> (47.3263, 19.8784)
  line L249 (47.3263, 19.8784) -> (47.3263, 18.6484)
  line L250 (47.3263, 18.6484) -> (47.3263, 17.4184)
  line L251 (47.3263, 17.4184) -> (47.6263, 17.4184)
  line L252 (47.6263, 17.4184) -> (47.9263, 17.4184)
  line L253 (47.9263, 17.4184) -> (47.9263, 19.1584)
  line L254 (47.9263, 19.1584) -> (47.9263, 20.8984)
  line L255 (47.9263, 20.8984) -> (47.7013, 20.8982)
  arc A840 (47.7013, 20.8982) -> (47.573, 20.8895) centre (47.702, 19.942) ccw
  arc A841 (47.573, 20.8895) -> (47.494, 20.8601) centre (47.5989, 20.6993) ccw
  arc A842 (47.494, 20.8601) -> (47.4311, 20.798) centre (47.6149, 20.6748) ccw
  arc A843 (47.4311, 20.798) -> (47.3563, 20.6732) centre (48.6359, 19.9903) ccw
  arc A844 (53.1019, 20.8234) -> (53.0616, 20.7671) centre (53.6963, 20.3555) ccw
  arc A845 (53.0616, 20.7671) -> (52.8904, 20.5023) centre (168.4936, -54.0893) ccw
  arc A846 (52.8904, 20.5023) -> (52.6905, 20.1908) centre (115.9975, -20.2168) ccw
  arc A847 (52.6905, 20.1908) -> (52.4646, 19.8356) centre (158.415, -47.2912) ccw
  line L256 (52.4646, 19.8356) -> (51.8863, 18.9229)
  line L257 (51.8863, 18.9229) -> (51.8863, 18.5306)
  line L258 (51.8863, 18.5306) -> (51.8863, 18.1384)
  line L259 (51.8863, 18.1384) -> (52.5463, 18.1384)
  line L260 (52.5463, 18.1384) -> (53.2063, 18.1384)
  line L261 (53.2063, 18.1384) -> (53.2063, 17.7784)
  line L262 (53.2063, 17.7784) -> (53.2063, 17.4184)
  line L263 (53.2063, 17.4184) -> (53.4763, 17.4184)
  line L264 (53.4763, 17.4184) -> (53.7463, 17.4184)
  line L265 (53.7463, 17.4184) -> (53.7463, 17.7784)
  line L266 (53.7463, 17.7784) -> (53.7463, 18.1384)
  line L267 (53.7463, 18.1384) -> (53.9263, 18.1384)
  arc A848 (53.9263, 18.1384) -> (54.0343, 18.1462) centre (53.9263, 18.8879) ccw
  arc A849 (54.0343, 18.1462) -> (54.0813, 18.1759) centre (54.0245, 18.2137) ccw
  arc A850 (54.0813, 18.1759) -> (54.1022, 18.2393) centre (53.9771, 18.2454) ccw
  arc A851 (54.1022, 18.2393) -> (54.1063, 18.4084) centre (50.6258, 18.4084) ccw
  arc A852 (54.1063, 18.4084) -> (54.1022, 18.5775) centre (50.6258, 18.4084) ccw
  arc A853 (54.1022, 18.5775) -> (54.0813, 18.6409) centre (53.9771, 18.5714) ccw
  arc A854 (54.0813, 18.6409) -> (54.0343, 18.6706) centre (54.0245, 18.6031) ccw
  arc A855 (54.0343, 18.6706) -> (53.9263, 18.6784) centre (53.9263, 17.9289) ccw
  line L268 (53.9263, 18.6784) -> (53.7463, 18.6784)
  line L269 (53.7463, 18.6784) -> (53.7463, 19.7884)
  line L270 (53.7463, 19.7884) -> (53.7463, 20.8984)
  line L271 (53.7463, 20.8984) -> (53.4536, 20.8984)
  arc A856 (53.4536, 20.8984) -> (53.3365, 20.8929) centre (53.4536, 19.6392) ccw
  arc A857 (53.3365, 20.8929) -> (53.2291, 20.8765) centre (53.423, 19.9674) ccw
  arc A858 (53.2291, 20.8765) -> (53.1431, 20.8527) centre (53.3825, 20.1571) ccw
  arc A859 (53.1431, 20.8527) -> (53.1019, 20.8234) centre (53.1722, 20.768) ccw
  arc A860 (53.1637, 18.7482) -> (53.1856, 18.7577) centre (53.1627, 18.7807) ccw
  arc A861 (53.0432, 18.7454) -> (53.1637, 18.7482) centre (52.9242, 26.2744) ccw
  arc A862 (52.9004, 18.7456) -> (53.0432, 18.7454) centre (52.9785, 22.8413) ccw
  arc A863 (52.7358, 18.7506) -> (52.9004, 18.7456) centre (53.0384, 25.9855) ccw
  line L272 (52.7358, 18.7506) -> (52.3108, 18.7684)
  line L273 (52.3108, 18.7684) -> (52.7435, 19.4284)
  line L274 (52.7435, 19.4284) -> (53.1763, 20.0884)
  line L275 (53.1763, 20.0884) -> (53.1934, 19.4355)
  arc A864 (53.1982, 19.1834) -> (53.1934, 19.4355) centre (35.9552, 18.9838) ccw
  arc A865 (53.1982, 18.9671) -> (53.1982, 19.1834) centre (43.813, 19.0748) ccw
  arc A866 (53.1953, 18.7806) -> (53.1982, 18.9671) centre (27.5538, 19.2612) ccw
  arc A867 (53.1856, 18.7577) -> (53.1953, 18.7806) centre (53.1621, 18.7812) ccw
  arc A868 (55.6288, 20.6906) -> (55.6663, 20.8165) centre (55.4362, 20.8165) ccw
  arc A869 (55.5124, 20.5509) -> (55.6288, 20.6906) centre (54.9721, 21.1197) ccw
  arc A870 (55.353, 20.4298) -> (55.5124, 20.5509) centre (54.8813, 21.2154) ccw
  arc A871 (55.1831, 20.3575) -> (55.353, 20.4298) centre (55.0096, 21.0017) ccw
  arc A872 (55.1831, 20.3575) -> (55.0449, 20.3139) centre (55.6238, 18.7209) ccw
  arc A873 (55.0449, 20.3139) -> (54.983, 20.2715) centre (55.0962, 20.1727) ccw
  arc A874 (54.983, 20.2715) -> (54.9542, 20.2076) centre (55.0742, 20.1919) ccw
  arc A875 (54.9542, 20.2076) -> (54.9463, 20.0861) centre (55.8841, 20.0861) ccw
  line L276 (54.9463, 20.0861) -> (54.9463, 19.8784)
  line L277 (54.9463, 19.8784) -> (55.2763, 19.8784)
  line L278 (55.2763, 19.8784) -> (55.6063, 19.8784)
  line L279 (55.6063, 19.8784) -> (55.6063, 18.6484)
  line L280 (55.6063, 18.6484) -> (55.6063, 17.4184)
  line L281 (55.6063, 17.4184) -> (55.8763, 17.4184)
  line L282 (55.8763, 17.4184) -> (56.1463, 17.4184)
  line L283 (56.1463, 17.4184) -> (56.1463, 19.1584)
  line L284 (56.1463, 19.1584) -> (56.1463, 20.8984)
  line L285 (56.1463, 20.8984) -> (55.9063, 20.8984)
  arc A876 (55.9063, 20.8984) -> (55.7987, 20.8938) centre (55.9063, 19.6496) ccw
  arc A877 (55.7987, 20.8938) -> (55.7252, 20.8783) centre (55.8255, 20.5846) ccw
  arc A878 (55.7252, 20.8783) -> (55.682, 20.8524) centre (55.7644, 20.7636) ccw
  arc A879 (55.682, 20.8524) -> (55.6663, 20.8165) centre (55.7153, 20.8165) ccw
  arc A880 (61.022, 20.556) -> (61.0963, 20.6732) centre (60.2725, 21.1129) ccw
  arc A881 (60.9434, 20.4762) -> (61.022, 20.556) centre (60.6972, 20.7973) ccw
  arc A882 (60.8411, 20.4167) -> (60.9434, 20.4762) centre (60.6603, 20.8455) ccw
  arc A883 (60.6913, 20.3628) -> (60.8411, 20.4167) centre (60.2646, 21.7837) ccw
  arc A884 (60.6913, 20.3628) -> (60.5212, 20.3062) centre (61.5526, 17.4944) ccw
  arc A885 (60.5212, 20.3062) -> (60.4492, 20.2601) centre (60.5896, 20.1196) ccw
  arc A886 (60.4492, 20.2601) -> (60.4159, 20.1955) centre (60.5332, 20.1761) ccw
  arc A887 (60.4159, 20.1955) -> (60.4063, 20.0778) centre (61.1274, 20.0778) ccw
  line L286 (60.4063, 20.0778) -> (60.4063, 19.8784)
  line L287 (60.4063, 19.8784) -> (60.7363, 19.8784)
  line L288 (60.7363, 19.8784) -> (61.0663, 19.8784)
  line L289 (61.0663, 19.8784) -> (61.0663, 18.6484)
  line L290 (61.0663, 18.6484) -> (61.0663, 17.4184)
  line L291 (61.0663, 17.4184) -> (61.3663, 17.4184)
  line L292 (61.3663, 17.4184) -> (61.6663, 17.4184)
  line L293 (61.6663, 17.4184) -> (61.6663, 19.1584)
  line L294 (61.6663, 19.1584) -> (61.6663, 20.8984)
  line L295 (61.6663, 20.8984) -> (61.4413, 20.8982)
  arc A888 (61.4413, 20.8982) -> (61.313, 20.8895) centre (61.442, 19.942) ccw
  arc A889 (61.313, 20.8895) -> (61.234, 20.8601) centre (61.3389, 20.6993) ccw
  arc A890 (61.234, 20.8601) -> (61.1711, 20.798) centre (61.3549, 20.6748) ccw
  arc A891 (61.1711, 20.798) -> (61.0963, 20.6732) centre (62.3759, 19.9903) ccw
  line L296 (17.0263, 20.4484) -> (17.0263, 20.1784)
  line L297 (17.0263, 20.1784) -> (17.4763, 20.1784)
  line L298 (17.4763, 20.1784) -> (17.9263, 20.1784)
  line L299 (17.9263, 20.1784) -> (17.9263, 19.0984)
  line L300 (17.9263, 19.0984) -> (17.9263, 18.0184)
  line L301 (17.9263, 18.0184) -> (17.3863, 18.0184)
  line L302 (17.3863, 18.0184) -> (16.8463, 18.0184)
  line L303 (16.8463, 18.0184) -> (16.8463, 17.7484)
  line L304 (16.8463, 17.7484) -> (16.8463, 17.4784)
  line L305 (16.8463, 17.4784) -> (18.2563, 17.4784)
  line L306 (18.2563, 17.4784) -> (19.6663, 17.4784)
  line L307 (19.6663, 17.4784) -> (19.6663, 17.7461)
  line L308 (19.6663, 17.7461) -> (19.6663, 18.0139)
  line L309 (19.6663, 18.0139) -> (19.1113, 18.0311)
  line L310 (19.1113, 18.0311) -> (18.5563, 18.0484)
  line L311 (18.5563, 18.0484) -> (18.5399, 19.1134)
  line L312 (18.5399, 19.1134) -> (18.5235, 20.1784)
  line L313 (18.5235, 20.1784) -> (19.0049, 20.1784)
  line L314 (19.0049, 20.1784) -> (19.4863, 20.1784)
  line L315 (19.4863, 20.1784) -> (19.4863, 20.4484)
  line L316 (19.4863, 20.4484) -> (19.4863, 20.7184)
  line L317 (19.4863, 20.7184) -> (18.2563, 20.7184)
  line L318 (18.2563, 20.7184) -> (17.0263, 20.7184)
  line L319 (17.0263, 20.7184) -> (17.0263, 20.4484)
  arc A892 (20.5522, 18.8217) -> (20.5659, 19.3534) centre (10.1156, 19.3584) ccw
  arc A893 (20.5055, 18.4665) -> (20.5522, 18.8217) centre (18.2909, 18.9379) ccw
  arc A894 (20.4122, 18.1786) -> (20.5055, 18.4665) centre (19.0759, 18.7708) ccw
  arc A895 (20.2523, 17.8797) -> (20.4122, 18.1786) centre (18.3208, 19.1055) ccw
  line L320 (20.2523, 17.8797) -> (20.0691, 17.5911)
  line L321 (20.0691, 17.5911) -> (20.299, 17.3557)
  arc A896 (20.299, 17.3557) -> (20.4426, 17.2137) centre (24.3935, 21.3538) ccw
  arc A897 (20.4426, 17.2137) -> (20.511, 17.1695) centre (20.5921, 17.3704) ccw
  arc A898 (20.511, 17.1695) -> (20.5676, 17.1715) centre (20.5371, 17.2343) ccw
  arc A899 (20.5676, 17.1715) -> (20.6378, 17.2188) centre (20.437, 17.4407) ccw
  arc A900 (20.6378, 17.2188) -> (20.7628, 17.3735) centre (20.2066, 17.6953) ccw
  arc A901 (20.7628, 17.3735) -> (20.905, 17.6469) centre (17.7919, 19.0924) ccw
  arc A902 (20.905, 17.6469) -> (21.0276, 17.9466) centre (17.7598, 19.1073) ccw
  arc A903 (21.0276, 17.9466) -> (21.0939, 18.2011) centre (19.5886, 18.4577) ccw
  line L322 (21.0939, 18.2011) -> (21.1395, 18.4684)
  line L323 (21.1395, 18.4684) -> (22.0829, 18.4849)
  arc A904 (22.613, 18.4913) -> (22.0829, 18.4849) centre (22.9296, -29.8619) ccw
  arc A905 (22.8594, 18.4823) -> (22.613, 18.4913) centre (22.6318, 15.6198) ccw
  arc A906 (22.9893, 18.4589) -> (22.8594, 18.4823) centre (22.8065, 17.817) ccw
  arc A907 (23.0263, 18.4099) -> (22.9893, 18.4589) centre (22.9754, 18.4099) ccw
  arc A908 (23.0263, 18.4099) -> (23.0438, 18.3665) centre (23.0887, 18.4099) ccw
  arc A909 (23.0438, 18.3665) -> (23.0904, 18.338) centre (23.1223, 18.4423) ccw
  arc A910 (23.0904, 18.338) -> (23.1773, 18.3225) centre (23.1978, 18.6897) ccw
  arc A911 (23.1773, 18.3225) -> (23.3263, 18.3184) centre (23.3263, 21.0007) ccw
  line L324 (23.3263, 18.3184) -> (23.6263, 18.3184)
  line L325 (23.6263, 18.3184) -> (23.6263, 19.1884)
  line L326 (23.6263, 19.1884) -> (23.6263, 20.0584)
  line L327 (23.6263, 20.0584) -> (22.0963, 20.0584)
  line L328 (22.0963, 20.0584) -> (20.5663, 20.0584)
  line L329 (20.5663, 20.0584) -> (20.5659, 19.3534)
  line L330 (23.0263, 19.2484) -> (23.0263, 18.9784)
  line L331 (23.0263, 18.9784) -> (22.0963, 18.9784)
  line L332 (22.0963, 18.9784) -> (21.1663, 18.9784)
  line L333 (21.1663, 18.9784) -> (21.1663, 19.2484)
  line L334 (21.1663, 19.2484) -> (21.1663, 19.5184)
  line L335 (21.1663, 19.5184) -> (22.0963, 19.5184)
  line L336 (22.0963, 19.5184) -> (23.0263, 19.5184)
  line L337 (23.0263, 19.5184) -> (23.0263, 19.2484)
  line L338 (7.5463, 19.2184) -> (7.5463, 18.4984)
  line L339 (7.5463, 18.4984) -> (8.1463, 18.4984)
  line L340 (8.1463, 18.4984) -> (8.7463, 18.4984)
  line L341 (8.7463, 18.4984) -> (8.7463, 18.1504)
  arc A912 (8.7325, 17.9004) -> (8.7463, 18.1504) centre (6.4757, 18.1504) ccw
  arc A913 (8.6827, 17.7587) -> (8.7325, 17.9004) centre (8.4013, 17.9371) ccw
  arc A914 (8.5881, 17.684) -> (8.6827, 17.7587) centre (8.5291, 17.8561) ccw
  arc A915 (8.4343, 17.6584) -> (8.5881, 17.684) centre (8.4343, 18.1326) ccw
  arc A916 (8.4343, 17.6584) -> (8.3104, 17.6526) centre (8.4343, 16.3316) ccw
  arc A917 (8.3104, 17.6526) -> (8.2783, 17.6247) centre (8.3138, 17.6162) ccw
  arc A918 (8.2783, 17.6247) -> (8.2818, 17.5682) centre (8.3721, 17.6023) ccw
  arc A919 (8.2818, 17.5682) -> (8.3628, 17.3596) centre (18.4558, 21.398) ccw
  arc A920 (8.3628, 17.3596) -> (8.43, 17.2112) centre (10.0695, 18.0425) ccw
  arc A921 (8.43, 17.2112) -> (8.4859, 17.1505) centre (8.5653, 17.2798) ccw
  arc A922 (8.4859, 17.1505) -> (8.5685, 17.1243) centre (8.5799, 17.3035) ccw
  arc A923 (8.5685, 17.1243) -> (8.7555, 17.1184) centre (8.7555, 20.0816) ccw
  arc A924 (8.7555, 17.1184) -> (8.9113, 17.1254) centre (8.7555, 18.8574) ccw
  arc A925 (8.9113, 17.1254) -> (9.0215, 17.1483) centre (8.8676, 17.6118) ccw
  arc A926 (9.0215, 17.1483) -> (9.1109, 17.1926) centre (8.9082, 17.4893) ccw
  arc A927 (9.1109, 17.1926) -> (9.199, 17.2657) centre (8.7636, 17.7011) ccw
  arc A928 (9.199, 17.2657) -> (9.2804, 17.3685) centre (8.7989, 17.6658) ccw
  arc A929 (9.2804, 17.3685) -> (9.3231, 17.4751) centre (8.994, 17.5453) ccw
  arc A930 (9.3231, 17.4751) -> (9.3419, 17.6329) centre (8.4744, 17.6562) ccw
  arc A931 (9.3419, 17.6329) -> (9.3463, 17.9557) centre (-2.6677, 17.9557) ccw
  line L342 (9.3463, 17.9557) -> (9.3463, 18.4984)
  line L343 (9.3463, 18.4984) -> (9.8863, 18.4984)
  line L344 (9.8863, 18.4984) -> (10.4263, 18.4984)
  line L345 (10.4263, 18.4984) -> (10.4263, 19.2184)
  line L346 (10.4263, 19.2184) -> (10.4263, 19.9384)
  line L347 (10.4263, 19.9384) -> (8.9863, 19.9384)
  line L348 (8.9863, 19.9384) -> (7.5463, 19.9384)
  line L349 (7.5463, 19.9384) -> (7.5463, 19.2184)
  arc A932 (9.7952, 19.157) -> (9.8155, 19.2334) centre (9.7149, 19.2191) ccw
  arc A933 (9.7255, 19.1155) -> (9.7952, 19.157) centre (9.7077, 19.2247) ccw
  arc A934 (9.5519, 19.1006) -> (9.7255, 19.1155) centre (9.5429, 20.2318) ccw
  arc A935 (8.9905, 19.0984) -> (9.5519, 19.1006) centre (8.9904, 89.2475) ccw
  line L350 (8.9905, 19.0984) -> (8.1463, 19.0984)
  line L351 (8.1463, 19.0984) -> (8.1463, 19.2501)
  line L352 (8.1463, 19.2501) -> (8.1463, 19.4018)
  line L353 (8.1463, 19.4018) -> (8.9713, 19.3851)
  arc A936 (9.5036, 19.3717) -> (8.9713, 19.3851) centre (7.8747, -34.809) ccw
  arc A937 (9.6879, 19.3525) -> (9.5036, 19.3717) centre (9.4659, 18.1172) ccw
  arc A938 (9.7741, 19.3106) -> (9.6879, 19.3525) centre (9.6567, 19.1787) ccw
  arc A939 (9.8155, 19.2334) -> (9.7741, 19.3106) centre (9.6894, 19.2155) ccw
  arc A940 (15.8926, 19.7152) -> (15.8067, 19.5774) centre (19.6459, 17.2823) ccw
  arc A941 (15.8067, 19.5774) -> (15.7858, 19.517) centre (15.9414, 19.4968) ccw
  arc A942 (15.7858, 19.517) -> (15.8, 19.4745) centre (15.8366, 19.5104) ccw
  arc A943 (15.8, 19.4745) -> (15.8558, 19.431) centre (15.9901, 19.6605) ccw
  arc A944 (15.9147, 19.395) -> (15.8558, 19.431) centre (14.9274, 17.8444) ccw
  arc A945 (16.0155, 19.3302) -> (15.9147, 19.395) centre (7.8762, 6.7694) ccw
  arc A946 (16.1318, 19.2542) -> (16.0155, 19.3302) centre (6.9883, 5.3992) ccw
  arc A947 (16.2493, 19.176) -> (16.1318, 19.2542) centre (6.3635, 4.4524) ccw
  line L354 (16.2493, 19.176) -> (16.5359, 18.9835)
  line L355 (16.5359, 18.9835) -> (16.6911, 19.187)
  arc A948 (16.6911, 19.187) -> (16.7505, 19.2692) centre (15.137, 20.3723) ccw
  arc A949 (16.7505, 19.2692) -> (16.8007, 19.3481) centre (15.5872, 20.0645) ccw
  arc A950 (16.8007, 19.3481) -> (16.838, 19.4158) centre (15.6575, 20.023) ccw
  arc A951 (16.838, 19.4158) -> (16.8463, 19.4498) centre (16.7719, 19.4498) ccw
  arc A952 (16.8463, 19.4498) -> (16.811, 19.5168) centre (16.765, 19.4498) ccw
  arc A953 (16.811, 19.5168) -> (16.5092, 19.7187) centre (8.1493, 6.8996) ccw
  arc A954 (16.5092, 19.7187) -> (16.2094, 19.9073) centre (10.6327, 10.7076) ccw
  arc A955 (16.2094, 19.9073) -> (16.0982, 19.9377) centre (16.1007, 19.7279) ccw
  arc A956 (16.0982, 19.9377) -> (16.0661, 19.9251) centre (16.0987, 19.8888) ccw
  arc A957 (16.0661, 19.9251) -> (16.0122, 19.872) centre (16.6153, 19.3146) ccw
  arc A958 (16.0122, 19.872) -> (15.9521, 19.8002) centre (16.7115, 19.2257) ccw
  arc A959 (15.9521, 19.8002) -> (15.8926, 19.7152) centre (17.0934, 18.9368) ccw
  line L356 (49.2463, 19.0984) -> (49.2463, 18.8584)
  line L357 (49.2463, 18.8584) -> (50.2063, 18.8584)
  line L358 (50.2063, 18.8584) -> (51.1663, 18.8584)
  line L359 (51.1663, 18.8584) -> (51.1663, 19.0984)
  line L360 (51.1663, 19.0984) -> (51.1663, 19.3384)
  line L361 (51.1663, 19.3384) -> (50.2063, 19.3384)
  line L362 (50.2063, 19.3384) -> (49.2463, 19.3384)
  line L363 (49.2463, 19.3384) -> (49.2463, 19.0984)
  line L364 (57.4663, 19.0984) -> (57.4663, 18.8584)
  line L365 (57.4663, 18.8584) -> (58.4263, 18.8584)
  line L366 (58.4263, 18.8584) -> (59.3863, 18.8584)
  line L367 (59.3863, 18.8584) -> (59.3863, 19.0984)
  line L368 (59.3863, 19.0984) -> (59.3863, 19.3384)
  line L369 (59.3863, 19.3384) -> (58.4263, 19.3384)
  line L370 (58.4263, 19.3384) -> (57.4663, 19.3384)
  line L371 (57.4663, 19.3384) -> (57.4663, 19.0984)
  arc A960 (16.1895, 18.2911) -> (16.2535, 18.445) centre (14.4975, 19.0853) ccw
  arc A961 (16.1019, 18.1174) -> (16.1895, 18.2911) centre (13.0609, 19.7595) ccw
  arc A962 (16.006, 17.9512) -> (16.1019, 18.1174) centre (13.1135, 19.7311) ccw
  arc A963 (15.9165, 17.8209) -> (16.006, 17.9512) centre (14.6657, 18.7759) ccw
  line L372 (15.9165, 17.8209) -> (15.707, 17.5465)
  line L373 (15.707, 17.5465) -> (15.9303, 17.3625)
  arc A964 (15.9303, 17.3625) -> (16.0193, 17.292) centre (17.788, 19.6161) ccw
  arc A965 (16.0193, 17.292) -> (16.102, 17.2325) centre (17.1667, 18.7998) ccw
  arc A966 (16.102, 17.2325) -> (16.1725, 17.1866) centre (17.2845, 18.9731) ccw
  arc A967 (16.1725, 17.1866) -> (16.2013, 17.1784) centre (16.2013, 17.2328) ccw
  arc A968 (16.2013, 17.1784) -> (16.2776, 17.2201) centre (16.2013, 17.2692) ccw
  arc A969 (16.2776, 17.2201) -> (16.4411, 17.4871) centre (10.4204, 20.9885) ccw
  arc A970 (16.4411, 17.4871) -> (16.6029, 17.7912) centre (12.4957, 19.7815) ccw
  arc A971 (16.6029, 17.7912) -> (16.7292, 18.0861) centre (13.5102, 19.2899) ccw